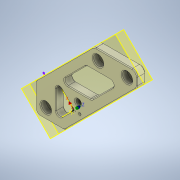
# Autodesk Inventor part: NEW_ACU_FIX2
Saved by Autodesk Inventor 2022 (Build 260153000, 153)
## iProperties
Created: 2021-11-12
Part Number: NEW_ACU_FIX2
Material: Generic
Document SubType Name: Modeling
Designer: Viktor
Density: 1 g/cm^3
Appearance: Default
Author: Viktor
Autodesk Inventor part; units mm, degrees
ref_plane "YZ Plane" through (0, 0, 0) normal (1, 0, 0) x (0, 1, 0)
ref_plane "XZ Plane" through (0, 0, 0) normal (0, 1, 0) x (-1, 0, 0)
ref_plane "XY Plane" through (0, 0, 0) normal (0, 0, 1) x (1, 0, 0)
sketch "Sketch1" plane through (0, 0, 0) normal (0, 0, 1) x (1, 0, 0)
  line L0 (0, 0) -> (0, -56.5685)
  line L1 (0, -56.5685) -> (113.4706, 56.902)
  line L2 (113.4706, 56.902) -> (56.902, 56.902)
  line L3 (56.902, 56.902) -> (0, 0)
  line L4 (-0.4955, 36.902) -> (119.5045, 36.902) construction
  circle A0 centre (89.3284, 46.902) radius 2.25
  circle A1 centre (61.0442, 46.902) radius 2.25
  line L5 (61.0442, 46.902) -> (89.3284, 46.902) construction
  line L6 (20, 35.2608) -> (20, -60.0641) construction
  circle A2 centre (10, -18.2843) radius 2.25
  circle A3 centre (41.5, 1.902) radius 2.75
  dimension "d1" = 40
  dimension "d2" = 20
  dimension "d3" = 10
  dimension "d4" = 4.5
  dimension "d5" = 4.5
  dimension "d6" = 4.5
  dimension "d8" = 5.5
  dimension "d9" = 41.5
  dimension "d10" = 12
  dimension "d11" = 35
  dimension "d12" = 10
  dimension "d14" = 10
  dimension "d17" = 20
  dimension "d18" = 10
  dimension "d19" = 20
  dimension "d20" = 135
  constraints: 14 end point, 4 centre point, 2 horizontal, 2 vertical, 1 parallel, 1 perpendicular
  measures "d1" distance between parallel lines of L1 L3
  measures "d2" distance between parallel lines of L2 L4
  measures "d3" distance between parallel lines of L2 L5
  measures "d4" diameter of A0
  measures "d5" diameter of A1
  measures "d6" diameter of A2
  measures "d8" diameter of A3
  measures "d9" distance from line of L0 A3.centre
  measures "d10" distance from line of L1 A3.centre
  measures "d11" distance from line of L4 A3.centre
  measures "d12" distance from line of L5.end L1
  measures "d14" distance from line of L3 L5.start
  measures "d17" distance between parallel lines of L6 L0
  measures "d18" distance from line of L6 A2.centre
  measures "d19" distance from line of L3 A2.centre
  measures "d20" angle of L0 L1
extrude "Extrusion1" add sketch "Sketch1" along normal blind 8
sketch "Sketch2" plane through (0, 0, 8) normal (0, 0, 1) x (1, 0, 0)
  line L0 (0, -56.5685) -> (113.4706, 56.902) projected
  line L1 (113.4706, 56.902) -> (56.902, 56.902) projected
  line L2 (56.902, 56.902) -> (0, 0) projected
  line L3 (0, 0) -> (0, -56.5685) projected
  circle A0 centre (41.5, 1.902) radius 2.75 projected
  circle A1 centre (10, -18.2843) radius 2.25 projected
  circle A2 centre (61.0442, 46.902) radius 2.25 projected
  circle A3 centre (89.3284, 46.902) radius 2.25 projected
  line L4 (0, -28.2843) -> (28.2843, -28.2843)
  line L5 (99.3284, 56.902) -> (99.3284, 42.7599)
  dimension "d25" = 10
  dimension "d26" = 10
  dimension "d27" = 10
  dimension "d28" = 10
  constraints: 4 end point, 3 point on line, 1 horizontal, 1 midpoint, 1 perpendicular
  measures "d25" distance from line of L3 A1.centre
  measures "d26" distance from line of A1.centre L4
  measures "d27" distance from line of L1 A3.centre
  measures "d28" distance from line of L5 A3.centre
extrude "Extrusion2" cut sketch "Sketch2" against normal through all contours L3 L4 L0 | L5 L1 L0
sketch "Sketch3" plane through (0, 0, 8) normal (0, 0, 1) x (1, 0, 0)
  line L0 (56.902, 56.902) -> (0, 0) projected
  line L1 (99.3284, 56.902) -> (56.902, 56.902) projected
  line L2 (49.6299, 36.902) -> (80.7426, 36.902)
  line L3 (80.7426, 36.902) -> (54.7426, 10.902)
  line L4 (54.7426, 10.902) -> (23.6299, 10.902)
  line L5 (23.6299, 10.902) -> (49.6299, 36.902)
  line L6 (28.2843, -28.2843) -> (99.3284, 42.7599) projected
  circle A0 centre (41.5, 1.902) radius 2.75 projected
  circle A1 centre (61.0442, 46.902) radius 2.25 projected
  dimension "d31" = 9
  dimension "d32" = 9
  dimension "d33" = 20
  dimension "d34" = 9
  dimension "d35" = 10
  constraints: 8 end point, 4 parallel, 1 horizontal
  measures "d31" distance between parallel lines of L0 L5
  measures "d32" distance between parallel lines of L6 L3
  measures "d33" distance between parallel lines of L1 L2
  measures "d34" distance from line of A0.centre L4
  measures "d35" distance from line of A1.centre L2
extrude "Extrusion3" cut sketch "Sketch3" against normal through all contours L2 L3 L4 L5
sketch "Sketch4" plane through (0, 0, 8) normal (0, 0, 1) x (1, 0, 0)
  line L0 (20, 1) -> (20, -23.8406)
  line L1 (20, -23.8406) -> (37.2574, -6.5833)
  line L2 (37.2574, -6.5833) -> (21.701, 8.9731)
  line L3 (0, 0) -> (0, -28.2843) projected
  line L4 (28.2843, -28.2843) -> (99.3284, 42.7599) projected
  line L5 (80.7426, 36.902) -> (54.7426, 10.902) projected
  line L6 (56.902, 56.902) -> (0, 0) projected
  line L7 (21.701, 8.9731) -> (20, 7.2721)
  line L8 (20, 7.2721) -> (20, 1)
  circle A0 centre (41.5, 1.902) radius 2.75 projected
  dimension "d39" = 20
  dimension "d41" = 9
  dimension "d42" = 9
  dimension "d43" = 9
  dimension "d44" = 90
  dimension "d45" = 9
  dimension "d46" = 90
  constraints: 10 end point, 1 collinear, 1 parallel, 1 vertical
  measures "d39" distance between parallel lines of L3 L0
  measures "d41" distance between parallel lines of L4 L1
  measures "d42" distance between parallel lines of L4 L5
  measures "d43" distance from line of L6 L2.end
  measures "d44" angle of L2 L1
  measures "d45" distance from line of A0.centre L2
  measures "d46" angle of L2 L7
extrude "Extrusion4" cut sketch "Sketch4" against normal through all contours L8 L7 L2 L1 L0
sketch "Sketch5" plane through (0, 0, 8) normal (0, 0, 1) x (1, 0, 0)
  circle A0 centre (10, -18.2843) radius 2.25 projected
  circle A1 centre (41.5, 1.902) radius 2.75 projected
  circle A2 centre (61.0442, 46.902) radius 2.25 projected
  circle A3 centre (89.3284, 46.902) radius 2.25 projected
  circle A4 centre (10, -18.2843) radius 5
  circle A5 centre (61.0442, 46.902) radius 5
  circle A6 centre (89.3284, 46.902) radius 5
  point P0 (0, 0)
  dimension "d49" = 10
  dimension "d50" = 10
  dimension "d51" = 10
  constraints: 3 centre point, 3 coincident
  measures "d49" diameter of A5
  measures "d50" diameter of A6
  measures "d51" diameter of A4
extrude "Extrusion5" cut sketch "Sketch5" against normal blind 5.5 contours A2 | A4 | A5 | A6
sketch "Sketch6" plane through (0, 0, 0) normal (0, 0, -1) x (-1, 0, 0)
  circle A0 centre (-41.5, 1.902) radius 2.75 projected
  line L0 (-44.9293, -1.5273) -> (-46.1845, 3.1572)
  line L1 (-46.1845, 3.1572) -> (-42.7552, 6.5865)
  line L2 (-42.7552, 6.5865) -> (-38.0707, 5.3313)
  line L3 (-38.0707, 5.3313) -> (-36.8155, 0.6468)
  line L4 (-36.8155, 0.6468) -> (-40.2448, -2.7825)
  line L5 (-40.2448, -2.7825) -> (-44.9293, -1.5273)
  line L6 (-37.2574, -6.5833) -> (-21.701, 8.9731) projected
  point P0 (0, 0)
  dimension "d54" = 8.4
  constraints: 12 end point, 1 coincident, 1 parallel, 13 other
  measures "d54" distance between parallel lines of L2 L5
extrude "Extrusion6" cut sketch "Sketch6" against normal blind 3.8
sketch "Sketch7" plane through (0, 0, 0) normal (0, 0, -1) x (-1, 0, 0)
  line L0 (-42.7552, 6.5865) -> (-38.0707, 5.3313) projected
  line L1 (-40.2448, -2.7825) -> (-44.9293, -1.5273) projected
  line L2 (-42.7552, 6.5865) -> (-40.2448, -2.7825) construction
  circle A0 centre (-40.5683, -1.5751) radius 1.25
  point P0 (0, 0)
  dimension "d57" = 2.5
  constraints: 2 end point, 1 point on line, 3 other
extrude "Extrusion7" cut sketch "Sketch7" against normal up to surface (3.8 mm away)
pattern_circular "Circular Pattern1" count 6 over 360 about axis through (41.5, 1.902, 0) along (0, 0, 1) of "Extrusion7"
fillet "Fillet1" radius 3.25 8 edges at (21.701, 8.9731, 4) (20, 7.2721, 4) (20, -23.8406, 4) (37.2574, -6.5833, 4) (54.7426, 10.902, 4) (80.7426, 36.902, 4) (49.6299, 36.902, 4) (23.6299, 10.902, 4)
fillet "Fillet2" radius 5 6 edges at (99.3284, 42.7599, 4) (99.3284, 56.902, 4) (56.902, 56.902, 4) (0, 0, 4) (0, -28.2843, 4) (28.2843, -28.2843, 4)
chamfer "Chamfer1" distance 0.75 angle 45 30 edges at (28.451, 28.451, 8) (0.3806, -0.1577, 8) (0, -12.6777, 8) (1.4645, -26.8198, 8) (15.6066, -28.2843, 8) (28.1266, -27.9037, 8) (63.8063, 7.2378, 8) (98.9478, 42.9175, 8) (99.3284, 48.3665, 8) (97.864, 55.4376, 8) (76.6508, 56.902, 8) (57.0597, 56.5214, 8) (5, -18.2843, 8) (30.2537, 0.4204, 8) (35.9112, -6.5833, 8) (30.2537, -13.5869, 8) (22.0063, -18.997, 8) (20, -6.5833, 8) (22.0063, 5.8305, 8) (38.75, 1.902, 8) (61.9363, 36.902, 8) (75.8991, 34.8957, 8) (65.4445, 21.6039, 8) (54.6402, 11.1494, 8) (42.4363, 10.902, 8) (28.4735, 12.9083, 8) (38.928, 26.2001, 8) (49.7324, 36.6546, 8) (56.0442, 46.902, 8) (84.3284, 46.902, 8)
sketch "Sketch8" plane through (0, 0, 8) normal (0, 0, 1) x (1, 0, 0)
  circle A0 centre (61.0442, 46.902) radius 5.75 projected
  circle A1 centre (89.3284, 46.902) radius 5.75 projected
  circle A2 centre (10, -18.2843) radius 5.75 projected
  circle A3 centre (41.5, 1.902) radius 3.5 projected
  arc A4 (75.7249, 30.8236) -> (72.8964, 37.652) centre (72.8964, 33.652) ccw projected
  arc A5 (35.4896, -9.4117) -> (35.4896, -3.7548) centre (32.6612, -6.5833) ccw projected
  point P0 (0, 0)
sketch "Sketch9" plane through (0, 0, 8) normal (0, 0, 1) x (1, 0, 0)
  circle A0 centre (52.1863, 23.902) radius 2
  circle A1 centre (27.9556, -6.5833) radius 2
  line L0 (20, -15.9944) -> (20, 2.8279) projected
  arc A2 (35.4896, -9.4117) -> (35.4896, -3.7548) centre (32.6612, -6.5833) ccw projected
  line L1 (19.25, 2.8279) -> (19.25, -15.9944) projected
  line L2 (29.178, 16.4501) -> (48.678, 35.9501) projected
  line L3 (75.1945, 31.3539) -> (55.6945, 11.8539) projected
  line L4 (50.9761, 36.902) -> (72.8964, 36.902) projected
  line L5 (53.3964, 10.902) -> (31.4761, 10.902) projected
  circle A3 centre (-5, -23.2843) radius 3.1887
  line L6 (0, -2.0711) -> (0, -23.2843) projected
  line L7 (5, -28.2843) -> (26.2132, -28.2843) projected
  point P0 (0, 0)
  dimension "d70" = 0
  dimension "d71" = 4.7056
  dimension "d72" = 8.7056
  dimension "d73" = 17.4112
  dimension "d74" = 4
  dimension "d75" = 4
  dimension "d76" = 11
  dimension "d77" = 22
  dimension "d78" = 26
  dimension "d79" = 13
  dimension "d80" = 4
  dimension "d95" = 5
  dimension "d96" = 5
  constraints: 3 centre point
  measures "d70" vertical distance of A2.centre A1.centre
  measures "d71" distance of A2.centre A1.centre
  measures "d72" distance from line of A1.centre L1
  measures "d74" radius of A2
  measures "d75" diameter of A1
  measures "d76" distance from line of L2 A0.centre
  measures "d77" distance between parallel lines of L2 L3
  measures "d78" distance between parallel lines of L4 L5
  measures "d79" distance from line of L5 A0.centre
  measures "d80" diameter of A0
  measures "d95" distance from line of L6 A3.centre
  measures "d96" distance from line of L7 A3.centre
sketch "Sketch10" plane through (0, 0, 8) normal (0, 0, 1) x (1, 0, 0)
  circle A0 centre (43.2678, -6.9368) radius 1.25
  line L0 (34.9593, -8.8814) -> (25.5481, -18.2925) projected
  line L1 (75.1945, 31.3539) -> (55.6945, 11.8539) projected
  line L2 (29.7487, -26.8198) -> (97.864, 41.2954) projected
  line L3 (25.5481, 5.126) -> (34.9593, -4.2852) projected
  point P0 (0, 0)
  dimension "d82" = 2.5
  dimension "d83" = 4.5
  dimension "d85" = 9
  dimension "d86" = 4
  constraints: 1 centre point
  measures "d82" diameter of A0
  measures "d83" distance from line of L0 A0.centre
  measures "d85" distance between parallel lines of L2 L0
  measures "d86" distance from line of L3 A0.centre
extrude "Extrusion8" cut sketch "Sketch10" against normal up to surface (8 mm away)
sketch "Sketch11" plane through (0, 0, 0) normal (0, 0, -1) x (-1, 0, 0)
  circle A0 centre (-43.2678, -6.9368) radius 1.25 projected
  arc A1 (-29.7487, -26.8198) -> (-26.2132, -28.2843) centre (-26.2132, -23.2843) ccw projected
  line L0 (-26.2132, -28.2843) -> (-5, -28.2843) projected
  arc A2 (-5, -28.2843) -> (0, -23.2843) centre (-5, -23.2843) ccw projected
  line L1 (0, -2.0711) -> (0, -23.2843) projected
  arc A3 (0, -2.0711) -> (-1.4645, 1.4645) centre (-5, -2.0711) ccw projected
  line L2 (-55.4376, 55.4376) -> (-1.4645, 1.4645) projected
  arc A4 (-55.4376, 55.4376) -> (-58.9731, 56.902) centre (-58.9731, 51.902) ccw projected
  line L3 (-94.3284, 56.902) -> (-58.9731, 56.902) projected
  arc A5 (-94.3284, 56.902) -> (-99.3284, 51.902) centre (-94.3284, 51.902) ccw projected
  line L4 (-99.3284, 51.902) -> (-99.3284, 44.831) projected
  arc A6 (-99.3284, 44.831) -> (-97.864, 41.2954) centre (-94.3284, 44.831) ccw projected
  line L5 (-29.7487, -26.8198) -> (-97.864, 41.2954) projected
  arc A7 (-37.6994, -0.2371) -> (-37.139, 1.8542) centre (-38.0229, 0.9703) ccw projected
  line L6 (-37.6994, -0.2371) -> (-39.3609, -1.8986) projected
  arc A8 (-41.4522, -2.4589) -> (-39.3609, -1.8986) centre (-40.5683, -1.5751) ccw projected
  line L7 (-41.4522, -2.4589) -> (-43.7219, -1.8508) projected
  arc A9 (-45.2528, -0.3199) -> (-43.7219, -1.8508) centre (-44.0454, -0.6434) ccw projected
  line L8 (-45.2528, -0.3199) -> (-45.861, 1.9498) projected
  arc A10 (-45.3006, 4.0411) -> (-45.861, 1.9498) centre (-44.9771, 2.8337) ccw projected
  line L9 (-45.3006, 4.0411) -> (-43.6391, 5.7026) projected
  arc A11 (-41.5478, 6.263) -> (-43.6391, 5.7026) centre (-42.4317, 5.3791) ccw projected
  line L10 (-41.5478, 6.263) -> (-39.2781, 5.6548) projected
  arc A12 (-37.7472, 4.1239) -> (-39.2781, 5.6548) centre (-38.9546, 4.4474) ccw projected
  line L11 (-37.7472, 4.1239) -> (-37.139, 1.8542) projected
  line L12 (-34.9593, -4.2852) -> (-25.5481, 5.126) projected
  arc A13 (-20, 2.8279) -> (-25.5481, 5.126) centre (-23.25, 2.8279) ccw projected
  line L13 (-20, 2.8279) -> (-20, -15.9944) projected
  arc A14 (-25.5481, -18.2925) -> (-20, -15.9944) centre (-23.25, -15.9944) ccw projected
  line L14 (-25.5481, -18.2925) -> (-34.9593, -8.8814) projected
  arc A15 (-34.9593, -4.2852) -> (-34.9593, -8.8814) centre (-32.6612, -6.5833) ccw projected
  line L15 (-55.6945, 11.8539) -> (-75.1945, 31.3539) projected
  arc A16 (-72.8964, 36.902) -> (-75.1945, 31.3539) centre (-72.8964, 33.652) ccw projected
  line L16 (-72.8964, 36.902) -> (-50.9761, 36.902) projected
  arc A17 (-48.678, 35.9501) -> (-50.9761, 36.902) centre (-50.9761, 33.652) ccw projected
  line L17 (-48.678, 35.9501) -> (-29.178, 16.4501) projected
  arc A18 (-31.4761, 10.902) -> (-29.178, 16.4501) centre (-31.4761, 14.152) ccw projected
  line L18 (-31.4761, 10.902) -> (-53.3964, 10.902) projected
  arc A19 (-55.6945, 11.8539) -> (-53.3964, 10.902) centre (-53.3964, 14.152) ccw projected
  circle A20 centre (-89.3284, 46.902) radius 2.25 projected
  circle A21 centre (-61.0442, 46.902) radius 2.25 projected
  circle A22 centre (-10, -18.2843) radius 2.25 projected
  line L19 (-53.5208, -3.0477) -> (-56.3492, -0.2193)
  line L20 (-56.3492, -0.2193) -> (-52.8137, 3.3162)
  line L21 (-52.8137, 3.3162) -> (-49.9853, 0.4878)
  line L22 (-49.9853, 0.4878) -> (-53.5208, -3.0477)
  point P0 (0, 0)
  dimension "d89" = 4
  dimension "d90" = 10
  dimension "d91" = 5
  constraints: 8 end point, 2 parallel, 2 point on line, 1 perpendicular
  measures "d89" distance between parallel lines of L20 L22
  measures "d90" distance from line of A0.centre L22
  measures "d91" distance between parallel lines of L19 L21
extrude "Extrusion9" cut sketch "Sketch11" against normal blind 1 contours L5 L20 L21 L22
fillet "Fillet3" radius 2 2 edges at (49.9853, 0.4878, 0.5) (52.8137, 3.3162, 0.5)
sketch "Sketch12" plane through (0, 0, 0) normal (0, 0, -1) x (-1, 0, 0)
  line L0 (-25.5481, -18.2925) -> (-34.9593, -8.8814) projected
  line L1 (-34.9593, -4.2852) -> (-25.5481, 5.126) projected
  line L2 (-34.9593, -8.8814) -> (-35.4896, -9.4117) projected
  line L3 (-34.9593, -8.8814) -> (-37.2574, -6.5833)
  line L4 (-37.2574, -6.5833) -> (-34.9593, -4.2852)
  point P0 (0, 0)
  constraints: 4 end point, 2 collinear, 1 coincident
sketch "Sketch13" plane through (0, 0, 3.8) normal (0, 0, -1) x (-1, 0, 0)
  circle A0 centre (-41.5, 1.902) radius 2.75 projected
  line L0 (-42.7552, 6.5865) -> (-38.0707, 5.3313)
  line L1 (-38.0707, 5.3313) -> (-36.8155, 0.6468)
  line L2 (-36.8155, 0.6468) -> (-40.2448, -2.7825)
  line L3 (-40.2448, -2.7825) -> (-44.9293, -1.5273)
  line L4 (-44.9293, -1.5273) -> (-46.1845, 3.1572)
  line L5 (-46.1845, 3.1572) -> (-42.7552, 6.5865)
  line L6 (-41.5478, 6.263) -> (-39.2781, 5.6548) projected
  point P0 (0, 0)
  point P1 (-40.413, 5.9589)
  constraints: 12 end point, 2 midpoint, 1 coincident, 13 other
sketch "Sketch14" plane through (0, 0, 0) normal (0, 0, -1) x (-1, 0, 0)
  line L0 (-29.7487, -26.8198) -> (-53.5208, -3.0477) projected
  line L1 (-56.3492, -0.2193) -> (-54.2279, 1.902) projected
  circle A0 centre (-43.2678, -6.9368) radius 1.25 projected
  point P0 (0, 0)
  point P1 (-31.4761, 10.902)
  dimension "d97" = 25.4519
  dimension "d98" = 14
  dimension "d99" = 4.5
  measures "d97" distance from line of point (-31.476, 10.902) L0
  measures "d98" distance from line of L1 A0.centre
  measures "d99" distance from line of L0 A0.centre
chamfer "Chamfer2" distance 0.75 angle 45 27 edges at (15.6066, -28.2843, 0) (1.4645, -26.8198, 0) (0, -12.6777, 0) (0.3806, -0.1577, 0) (28.451, 28.451, 0) (57.0597, 56.5214, 0) (76.6508, 56.902, 0) (97.864, 55.4376, 0) (99.3284, 48.3665, 0) (98.9478, 42.9175, 0) (77.1066, 20.5381, 0) (28.1266, -27.9037, 0) (41.6348, -14.9338, 0) (30.2537, 0.4204, 0) (22.0063, -18.997, 0) (35.9112, -6.5833, 0) (22.0063, 5.8305, 0) (20, -6.5833, 0) (30.2537, -13.5869, 0) (42.4363, 10.902, 0) (54.6402, 11.1494, 0) (65.4445, 21.6039, 0) (75.8991, 34.8957, 0) (61.9363, 36.902, 0) (49.7324, 36.6546, 0) (38.928, 26.2001, 0) (28.4735, 12.9083, 0)
sketch "Sketch15" plane through (0, 0, 8) normal (0, 0, 1) x (1, 0, 0)
  line L0 (34.9593, -8.8814) -> (37.2574, -6.5833)
  line L1 (37.2574, -6.5833) -> (34.9593, -4.2852)
  line L2 (25.5481, 5.126) -> (34.9593, -4.2852) projected
  line L3 (34.9593, -8.8814) -> (25.5481, -18.2925) projected
  point P0 (0, 0)
  point P1 (35.4896, -9.4117)
  point P2 (35.4896, -3.7548)
  constraints: 4 end point, 2 collinear, 1 coincident
sketch "Sketch16" plane through (0, 0, 0) normal (0, 0, -1) x (-1, 0, 0)
  circle A0 centre (0, 2) radius 0.879
  point P0 (0, 0)
  constraints: 1 centre point
equation "\"d4\" = d5"
equation "\"d6\" = d5"
equation "\"d12\" = d14"
equation "\"d19\" = 0.5 * d1"
equation "\"d26\" = d25"
equation "\"d28\" = d27"
equation "\"d32\" = d31"
equation "\"d34\" = d31"
equation "\"d41\" = d42"
equation "\"d43\" = d41"
equation "\"d45\" = d41"
equation "\"d51\" = d49"
equation "\"d83\" = 0.5 * d85"
equation "\"d72\" = 0.5 * d73"
equation "\"d76\" = 0.5 * d77"
equation "\"d79\" = 0.5 * d78"
equation "\"d80\" = d75"
body "Solid1"
